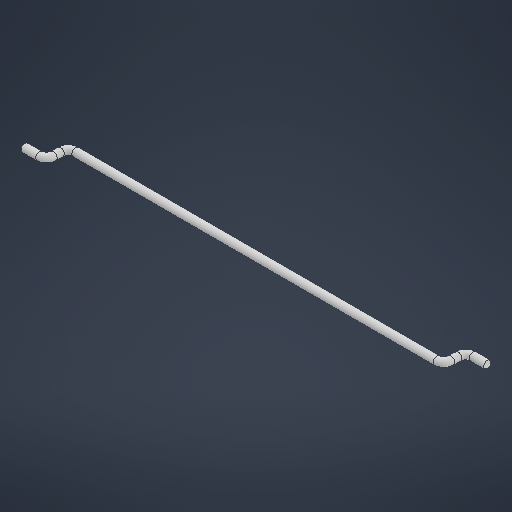
# Autodesk Inventor part: P_Wing_mid_servolink
Saved by Autodesk Inventor 2026 (Build 300175000, 175)
## iProperties
Created: 2025-09-02
Part Number: P_Wing_mid_servolink
Material: Generisch
Document SubType Name: Modeling
Designer: FAL
Density: 1 g/cm^3
Appearance: Vorgabe
Author: FAL
Autodesk Inventor part; units mm, degrees
ref_plane "YZ Plane" through (0, 0, 0) normal (1, 0, 0) x (0, 1, 0)
ref_plane "XZ Plane" through (0, 0, 0) normal (0, 1, 0) x (-1, 0, 0)
ref_plane "XY Plane" through (0, 0, 0) normal (0, 0, 1) x (1, 0, 0)
sketch "Skizze1" plane through (0, 0, 0) normal (0, 0, 1) x (1, 0, 0)
  line L0 (0, 0) -> (2, 0)
  line L1 (3, 1) -> (3, 2)
  line L2 (4, 3) -> (54, 3)
  line L3 (55, 4) -> (55, 5)
  line L4 (56, 6) -> (58, 6)
  arc A0 (2, 0) -> (3, 1) centre (2, 1) ccw
  arc A1 (4, 3) -> (3, 2) centre (4, 2) ccw
  arc A2 (54, 3) -> (55, 4) centre (54, 4) ccw
  arc A3 (56, 6) -> (55, 5) centre (56, 5) ccw
  dimension "d0" = 1
  dimension "d4" = 2
  dimension "d5" = 3
  dimension "d6" = 3
  dimension "d7" = 50
  dimension "d8" = 2
  constraints: 10 end point, 8 point on circle, 8 tangent, 4 centre point, 4 perpendicular, 3 equal radius, 1 horizontal
  measures "d0" radius of A0
  measures "d4" horizontal distance of L0.start A0.centre
  measures "d5" distance between parallel lines of L0 L2
  measures "d6" distance between parallel lines of L2 L4
  measures "d7" horizontal distance of A1.centre A2.centre
  measures "d8" horizontal distance of A3.centre L4.end
sketch "Skizze2" plane through (0, 0, 0) normal (1, 0, 0) x (0, 1, 0)
  circle A0 centre (0, 0) radius 0.5
  dimension "d1" = 1
  constraints: 1 centre point, 1 coincident
  measures "d1" diameter of A0
sweep "Sweeping1" add profiles "Skizze2" path "Skizze1" path curves L0 A0 L1 A1 L2 A2 L3 A3 L4
